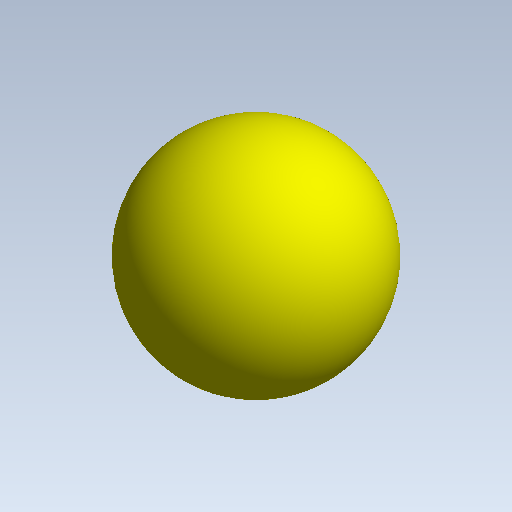
# Autodesk Inventor part: W 605-2Z_PART3
Saved by Autodesk Inventor 2020.2 (Build 242310000, 310)
## iProperties
Part Number: W 605-2Z_PART3
Material: Generic
Catalog Web Link: www.cadenas.de
Description: -Deep groove ball bearings
Vendor: SKF
Document SubType Name: Modeling
Designer: partserver
Manufacturer: SKF
Mass: 0.00706768 g
Surface Area: 0.178102 cm^2
Volume: 0.00706768 cm^3
Density: 1 g/cm^3
Appearance: PSOLRGB-192-192-192
Category: PARTsolutions
Company: SKF
PSOL_IDENT_0: {$CADENAS_DATA\23d-libs\skf\bearings_units_and_housings\ball_bearings\deep_groove_ball_bearings\bb1_
PSOL_IDENT_1: 001_101.prj},195 {VTYP=3D},{NB=W 605-2Z_PART3},{LINA=W 605-2Z_PART3},{NN=BB1_001_101_PART3},{NOPRJ=T
PSOL_IDENT_2: RUE},{DATE=26.02.2021 12:30:54},{GEOMDATE=05.02.2021 06:24:08},{VERSION=},{LINEID=16160},{WBVAR=},{W
PSOL_IDENT_3: BNUMERIC=}  {NB=W 605-2Z_PART3},{LINA=W 605-2Z_PART3},{KT=DUMMY},{DESIGNATION=W 605-2Z},{R12=0.20},{
PSOL_IDENT_4: DD=5.000},{D=14.000},{B=5.000},{C=},{CX=},{CXX=},{CA=0.000},{XXVARIANT=},{XXDESIGN=Single row stainl
PSOL_IDENT_5: ess steel},{XXSEALING=Shield on both sides},{DESIGN=dgbbw2z},{DESIGNIR=dgbbw2z},{VARIANT=},{DD1=7.79
PSOL_IDENT_6: },{DD2=6.9},{DD2X=},{DD2A=6.90},{D1=11.28},{D1X=MIN},{D2=12.2},{D2A=12.20},{D3=},{D3X=},{D3A=0.000},
PSOL_IDENT_7: {D4=},{HH=MIN},{BB=0.000},{BBX=},{BBA=0.000},{FF=},{R0MAX=MIN},{R0=MIN},{PITCH=9.50},{DW=2.381},{DDA
PSOL_IDENT_8: MIN=6.600},{DDAMAX=6.800},{DDBMIN=MIN},{DDBMAX=MIN},{DBMIN=MIN},{DAMAX=12.400},{BBAMIN=MIN},{CAMAX=M
PSOL_IDENT_9: IN},{RAMAX=0.200},{LOAD1=0.761},{LOAD2=0.260},{LOAD3=0.011},{SPEED1=110000},{SPEED2=53000},{KR=0.030
PSOL_IDENT_10: },{F0=6.600},{Z=7},{II=1},{MASS=0.003},{BEARING=W 605-2Z},{RING=},{HELP=1.360},{HELP2=0.900},{DD1ALG=
PSOL_IDENT_11: 3.895},{YALG=3.895},{PITCH1=9.500},{DW1=2.381},{YALG1=5.640},{HALG1=1.360},{SH=3.450},{CU=0.524},{HA
PSOL_IDENT_12: LG=1.395},{B1=0},{SHIELDHELP=2},{D4A=0.000},{FFA=0.000},{RS1=}
NB: W 605-2Z_PART3
NT: Deep groove ball bearings
NBSYN: $DESIGNATION._PART3
LINA: W 605-2Z_PART3
CATALOG: SKF
SUPPLIER: SKF
ARTICLENO: W 605-2Z_PART3
BOMINFO: W 605-2Z_PART3
CREATOR: CADENAS GmbH
Title: W 605-2Z_PART3
Author: Cadenas PARTsolutions
Comments: Deep groove ball bearings
Autodesk Inventor part; units mm, degrees
ref_plane "YZ Plane" through (0, 0, 0) normal (1, 0, 0) x (0, 1, 0)
ref_plane "XZ Plane" through (0, 0, 0) normal (0, 1, 0) x (-1, 0, 0)
ref_plane "XY Plane" through (0, 0, 0) normal (0, 0, 1) x (1, 0, 0)
sketch "Sketch_6" plane through (0, 0, 0) normal (0, 0, 1) x (1, 0, 0)
  line L0 (3.6905, 4.75) -> (1.3095, 4.75)
  arc A0 (3.6905, 4.75) -> (1.3095, 4.75) centre (2.5, 4.75) ccw
  line L1 (3.6905, 4.75) -> (1.3095, 4.75)
  dimension "d0" = 360
  constraints: 4 end point, 2 point on circle, 1 centre point
revolve "Revolution1" add sketch "Sketch_6" angle 360 about axis through (3.6905, 4.75, 0) along (1, 0, 0)
body "Solid1"
